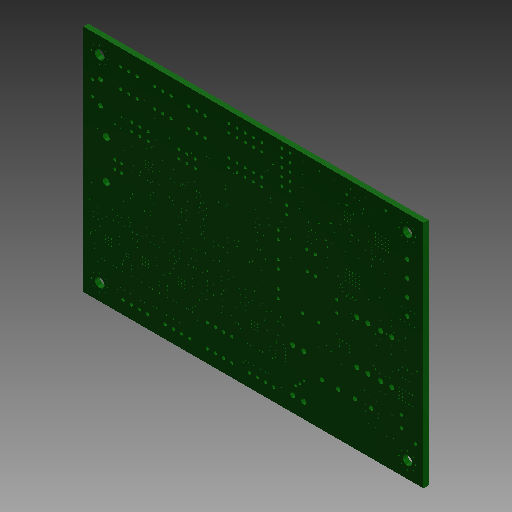
# Autodesk Inventor part: Mini-Rambo_Outline
Saved by Autodesk Inventor 2018.2 (Build 222227000, 227)
## iProperties
Part Number: Mini-Rambo_Outline
Material: Generic
Document SubType Name: Modeling
Designer: autocad
Appearance: Board Outline
Author: autocad
Autodesk Inventor part; units mm, degrees
ref_plane "YZ Plane" through (0, 0, 0) normal (1, 0, 0) x (0, 1, 0)
ref_plane "XZ Plane" through (0, 0, 0) normal (0, 1, 0) x (-1, 0, 0)
ref_plane "XY Plane" through (0, 0, 0) normal (0, 0, 1) x (1, 0, 0)
sketch "Sketch1" plane through (0, 0, 0) normal (0, 0, 1) x (1, 0, 0)
  line L0 (25, 25) -> (25, 96)
  line L1 (25, 96) -> (130, 96)
  line L2 (130, 96) -> (130, 25)
  line L3 (130, 25) -> (25, 25)
  circle A0 centre (93.0018, 43.156) radius 0.8001
  circle A1 centre (89.5982, 43.156) radius 0.8001
  circle A2 centre (89.5982, 29.694) radius 0.8001
  circle A3 centre (93.0018, 29.694) radius 0.8001
  circle A4 centre (109.4232, 60.556) radius 0.8001
  circle A5 centre (112.8268, 60.556) radius 0.8001
  circle A6 centre (112.8268, 47.094) radius 0.8001
  circle A7 centre (109.4232, 47.094) radius 0.8001
  circle A8 centre (116.7982, 47.119) radius 0.8001
  circle A9 centre (120.2018, 47.119) radius 0.8001
  circle A10 centre (120.2018, 60.581) radius 0.8001
  circle A11 centre (116.7982, 60.581) radius 0.8001
  circle A12 centre (69.89, 90.06) radius 0.45
  circle A13 centre (69.89, 92.6) radius 0.45
  circle A14 centre (72.43, 90.06) radius 0.45
  circle A15 centre (72.43, 92.6) radius 0.45
  circle A16 centre (74.97, 90.06) radius 0.45
  circle A17 centre (74.97, 92.6) radius 0.45
  circle A18 centre (77.51, 90.06) radius 0.45
  circle A19 centre (77.51, 92.6) radius 0.45
  circle A20 centre (80.05, 90.06) radius 0.45
  circle A21 centre (80.05, 92.6) radius 0.45
  circle A22 centre (69.84, 80.735) radius 0.45
  circle A23 centre (69.84, 83.275) radius 0.45
  circle A24 centre (72.38, 80.735) radius 0.45
  circle A25 centre (72.38, 83.275) radius 0.45
  circle A26 centre (74.92, 80.735) radius 0.45
  circle A27 centre (74.92, 83.275) radius 0.45
  circle A28 centre (77.46, 80.735) radius 0.45
  circle A29 centre (77.46, 83.275) radius 0.45
  circle A30 centre (80, 80.735) radius 0.45
  circle A31 centre (80, 83.275) radius 0.45
  circle A32 centre (63.19, 29) radius 0.508
  circle A33 centre (65.73, 29) radius 0.508
  circle A34 centre (68.27, 29) radius 0.508
  circle A35 centre (70.81, 29) radius 0.508
  circle A36 centre (63.19, 36) radius 0.508
  circle A37 centre (65.73, 36) radius 0.508
  circle A38 centre (68.27, 36) radius 0.508
  circle A39 centre (70.81, 36) radius 0.508
  circle A40 centre (27.7554, 83.2606) radius 0.508
  circle A41 centre (27.7554, 78.7394) radius 0.508
  circle A42 centre (30.2446, 84.5052) radius 0.7493
  circle A43 centre (30.2446, 77.4948) radius 0.7493
  circle A44 centre (57.46, 91) radius 0.508
  circle A45 centre (60, 91) radius 0.508
  circle A46 centre (62.54, 91) radius 0.508
  circle A47 centre (46.96, 91) radius 0.508
  circle A48 centre (49.5, 91) radius 0.508
  circle A49 centre (52.04, 91) radius 0.508
  circle A50 centre (36.46, 91) radius 0.508
  circle A51 centre (39, 91) radius 0.508
  circle A52 centre (41.54, 91) radius 0.508
  circle A53 centre (52.04, 85) radius 0.508
  circle A54 centre (49.5, 85) radius 0.508
  circle A55 centre (46.96, 85) radius 0.508
  circle A56 centre (62.54, 85) radius 0.508
  circle A57 centre (60, 85) radius 0.508
  circle A58 centre (57.46, 85) radius 0.508
  circle A59 centre (41.54, 85) radius 0.508
  circle A60 centre (39, 85) radius 0.508
  circle A61 centre (36.46, 85) radius 0.508
  circle A62 centre (85.1, 69.13) radius 0.508
  circle A63 centre (85.1, 71.67) radius 0.508
  circle A64 centre (85.1, 61.23) radius 0.508
  circle A65 centre (85.1, 63.77) radius 0.508
  circle A66 centre (87.7, 79.67) radius 0.508
  circle A67 centre (87.7, 77.13) radius 0.508
  circle A68 centre (94.13, 65.1) radius 0.508
  circle A69 centre (96.67, 65.1) radius 0.508
  circle A70 centre (85.1, 53.33) radius 0.508
  circle A71 centre (85.1, 55.87) radius 0.508
  circle A72 centre (88.765, 83.965) radius 0.45
  circle A73 centre (86.225, 83.965) radius 0.45
  circle A74 centre (88.765, 86.505) radius 0.45
  circle A75 centre (86.225, 86.505) radius 0.45
  circle A76 centre (88.765, 89.045) radius 0.45
  circle A77 centre (86.225, 89.045) radius 0.45
  circle A78 centre (88.765, 91.585) radius 0.45
  circle A79 centre (86.225, 91.585) radius 0.45
  circle A80 centre (88.765, 94.125) radius 0.45
  circle A81 centre (86.225, 94.125) radius 0.45
  circle A82 centre (32, 57.9802) radius 1.1049
  circle A83 centre (32, 70) radius 1.1049
  circle A84 centre (34.7178, 62.73) radius 0.4826
  circle A85 centre (34.7178, 65.25) radius 0.4826
  circle A86 centre (36.7244, 65.25) radius 0.4826
  circle A87 centre (36.7244, 62.73) radius 0.4826
  circle A88 centre (97.65, 53.2) radius 0.508
  circle A89 centre (92.65, 53.2) radius 0.508
  circle A90 centre (37.19, 29) radius 0.508
  circle A91 centre (39.73, 29) radius 0.508
  circle A92 centre (42.27, 29) radius 0.508
  circle A93 centre (44.81, 29) radius 0.508
  circle A94 centre (50.19, 29) radius 0.508
  circle A95 centre (52.73, 29) radius 0.508
  circle A96 centre (55.27, 29) radius 0.508
  circle A97 centre (57.81, 29) radius 0.508
  circle A98 centre (76.19, 29) radius 0.508
  circle A99 centre (78.73, 29) radius 0.508
  circle A100 centre (81.27, 29) radius 0.508
  circle A101 centre (83.81, 29) radius 0.508
  circle A102 centre (124.9934, 68.58) radius 0.6985
  circle A103 centre (124.9934, 73.66) radius 0.6985
  circle A104 centre (124.9934, 78.74) radius 0.6985
  circle A105 centre (124.9934, 83.82) radius 0.6985
  circle A106 centre (103.225, 62.103) radius 0.508
  circle A107 centre (103.225, 58.547) radius 0.508
  circle A108 centre (123.15, 37.722) radius 0.508
  circle A109 centre (123.15, 41.278) radius 0.508
  circle A110 centre (54.41, 75.376) radius 0.4826
  circle A111 centre (54.41, 77.916) radius 0.4826
  circle A112 centre (56.95, 75.376) radius 0.4826
  circle A113 centre (56.95, 77.916) radius 0.4826
  circle A114 centre (59.49, 75.376) radius 0.4826
  circle A115 centre (59.49, 77.916) radius 0.4826
  circle A116 centre (39.866, 75.376) radius 0.4826
  circle A117 centre (39.866, 77.916) radius 0.4826
  circle A118 centre (42.406, 75.376) radius 0.4826
  circle A119 centre (42.406, 77.916) radius 0.4826
  circle A120 centre (44.946, 75.376) radius 0.4826
  circle A121 centre (44.946, 77.916) radius 0.4826
  circle A122 centre (94, 70.9) radius 0.508
  circle A123 centre (96.54, 70.9) radius 0.508
  circle A124 centre (127.525, 35.7) radius 0.508
  circle A125 centre (123.222, 28.222) radius 0.1905
  circle A126 centre (126.778, 28.222) radius 0.1905
  circle A127 centre (126.778, 31.778) radius 0.1905
  circle A128 centre (123.222, 31.778) radius 0.1905
  circle A129 centre (122.46, 30) radius 0.1905
  circle A130 centre (127.54, 30) radius 0.1905
  circle A131 centre (125, 32.54) radius 0.1905
  circle A132 centre (125, 27.46) radius 0.1905
  circle A133 centre (28.222, 28.222) radius 0.1905
  circle A134 centre (31.778, 28.222) radius 0.1905
  circle A135 centre (31.778, 31.778) radius 0.1905
  circle A136 centre (28.222, 31.778) radius 0.1905
  circle A137 centre (27.46, 30) radius 0.1905
  circle A138 centre (32.54, 30) radius 0.1905
  circle A139 centre (30, 32.54) radius 0.1905
  circle A140 centre (30, 27.46) radius 0.1905
  circle A141 centre (28.222, 89.222) radius 0.1905
  circle A142 centre (31.778, 89.222) radius 0.1905
  circle A143 centre (31.778, 92.778) radius 0.1905
  circle A144 centre (28.222, 92.778) radius 0.1905
  circle A145 centre (27.46, 91) radius 0.1905
  circle A146 centre (32.54, 91) radius 0.1905
  circle A147 centre (30, 93.54) radius 0.1905
  circle A148 centre (30, 88.46) radius 0.1905
  circle A149 centre (123.222, 89.222) radius 0.1905
  circle A150 centre (126.778, 89.222) radius 0.1905
  circle A151 centre (126.778, 92.778) radius 0.1905
  circle A152 centre (123.222, 92.778) radius 0.1905
  circle A153 centre (122.46, 91) radius 0.1905
  circle A154 centre (127.54, 91) radius 0.1905
  circle A155 centre (125, 93.54) radius 0.1905
  circle A156 centre (125, 88.46) radius 0.1905
  circle A157 centre (98.605, 38.375) radius 0.6985
  circle A158 centre (103.685, 38.375) radius 0.6985
  circle A159 centre (108.765, 38.375) radius 0.6985
  circle A160 centre (113.845, 38.375) radius 0.6985
  circle A161 centre (97.625, 46.375) radius 0.1905
  circle A162 centre (101.45, 47.325) radius 0.1905
  circle A163 centre (99.95, 48.25) radius 0.1905
  circle A164 centre (86.075, 30.1) radius 0.1905
  circle A165 centre (84.375, 39.1) radius 0.1905
  circle A166 centre (84.5, 41.175) radius 0.1905
  circle A167 centre (87.375, 38.5) radius 0.1905
  circle A168 centre (87.375, 41.1437) radius 0.1905
  circle A169 centre (108.025, 59) radius 0.1905
  circle A170 centre (107.9, 60.775) radius 0.1905
  circle A171 centre (93.15, 35.35) radius 0.381
  circle A172 centre (91.775, 33.9) radius 0.381
  circle A173 centre (120.7, 33.775) radius 0.1905
  circle A174 centre (118.525, 33.2) radius 0.1905
  circle A175 centre (87.375, 40.2625) radius 0.1905
  circle A176 centre (87.375, 39.3813) radius 0.1905
  circle A177 centre (87.375, 37.6187) radius 0.1905
  circle A178 centre (125.725, 51.4) radius 0.1905
  circle A179 centre (124.525, 51.4) radius 0.1905
  circle A180 centre (123.5, 51.4) radius 0.1905
  circle A181 centre (95.325, 73.125) radius 0.1905
  circle A182 centre (94.3, 73.125) radius 0.1905
  circle A183 centre (94.45, 75.875) radius 0.1905
  circle A184 centre (96.8, 75.025) radius 0.1905
  circle A185 centre (96.8, 76.8) radius 0.1905
  circle A186 centre (95.425, 76.8) radius 0.1905
  circle A187 centre (94.3, 74.45) radius 0.1905
  circle A188 centre (88.95, 71.2) radius 0.1905
  circle A189 centre (89.05, 66.25) radius 0.1905
  circle A190 centre (99.85, 76.275) radius 0.3175
  circle A191 centre (115.15, 33.825) radius 0.1905
  circle A192 centre (113.075, 33.825) radius 0.1905
  circle A193 centre (112.175, 38.55) radius 0.1905
  circle A194 centre (58.4232, 78.8982) radius 0.1905
  circle A195 centre (71.375, 79.85) radius 0.1905
  circle A196 centre (117.2, 84.851) radius 0.1905
  circle A197 centre (117.2, 85.867) radius 0.1905
  circle A198 centre (117.2, 83.835) radius 0.1905
  circle A199 centre (117.2, 82.819) radius 0.1905
  circle A200 centre (116.184, 82.819) radius 0.1905
  circle A201 centre (115.168, 82.819) radius 0.1905
  circle A202 centre (115.168, 83.835) radius 0.1905
  circle A203 centre (116.184, 83.835) radius 0.1905
  circle A204 centre (116.184, 84.851) radius 0.1905
  circle A205 centre (115.168, 84.851) radius 0.1905
  circle A206 centre (115.168, 85.867) radius 0.1905
  circle A207 centre (116.184, 85.867) radius 0.1905
  circle A208 centre (118.216, 85.867) radius 0.1905
  circle A209 centre (119.232, 85.867) radius 0.1905
  circle A210 centre (119.232, 84.851) radius 0.1905
  circle A211 centre (118.216, 84.851) radius 0.1905
  circle A212 centre (118.216, 83.835) radius 0.1905
  circle A213 centre (119.232, 83.835) radius 0.1905
  circle A214 centre (119.232, 82.819) radius 0.1905
  circle A215 centre (118.216, 82.819) radius 0.1905
  circle A216 centre (109.116, 68.619) radius 0.1905
  circle A217 centre (110.132, 68.619) radius 0.1905
  circle A218 centre (110.132, 69.635) radius 0.1905
  circle A219 centre (109.116, 69.635) radius 0.1905
  circle A220 centre (109.116, 70.651) radius 0.1905
  circle A221 centre (110.132, 70.651) radius 0.1905
  circle A222 centre (110.132, 71.667) radius 0.1905
  circle A223 centre (109.116, 71.667) radius 0.1905
  circle A224 centre (107.084, 71.667) radius 0.1905
  circle A225 centre (106.068, 71.667) radius 0.1905
  circle A226 centre (106.068, 70.651) radius 0.1905
  circle A227 centre (107.084, 70.651) radius 0.1905
  circle A228 centre (107.084, 69.635) radius 0.1905
  circle A229 centre (106.068, 69.635) radius 0.1905
  circle A230 centre (106.068, 68.619) radius 0.1905
  circle A231 centre (107.084, 68.619) radius 0.1905
  circle A232 centre (108.1, 68.619) radius 0.1905
  circle A233 centre (108.1, 69.635) radius 0.1905
  circle A234 centre (108.1, 71.667) radius 0.1905
  circle A235 centre (108.1, 70.651) radius 0.1905
  circle A236 centre (45.212, 68.834) radius 0.1905
  circle A237 centre (45.212, 69.784) radius 0.1905
  circle A238 centre (44.2548, 69.7931) radius 0.1905
  circle A239 centre (44.267, 68.834) radius 0.1905
  circle A240 centre (44.262, 67.859) radius 0.1905
  circle A241 centre (45.212, 67.884) radius 0.1905
  circle A242 centre (46.162, 67.884) radius 0.1905
  circle A243 centre (46.162, 68.834) radius 0.1905
  circle A244 centre (46.162, 69.784) radius 0.1905
  circle A245 centre (32.7, 42.5706) radius 0.1905
  circle A246 centre (31.75, 42.5706) radius 0.1905
  circle A247 centre (31.7409, 41.6134) radius 0.1905
  circle A248 centre (32.7, 41.6256) radius 0.1905
  circle A249 centre (33.675, 41.6206) radius 0.1905
  circle A250 centre (33.65, 42.5706) radius 0.1905
  circle A251 centre (33.65, 43.5206) radius 0.1905
  circle A252 centre (32.7, 43.5206) radius 0.1905
  circle A253 centre (31.75, 43.5206) radius 0.1905
  circle A254 centre (44.153, 42.5706) radius 0.1905
  circle A255 centre (43.203, 42.5706) radius 0.1905
  circle A256 centre (43.1939, 41.6134) radius 0.1905
  circle A257 centre (44.153, 41.6256) radius 0.1905
  circle A258 centre (45.128, 41.6206) radius 0.1905
  circle A259 centre (45.103, 42.5706) radius 0.1905
  circle A260 centre (45.103, 43.5206) radius 0.1905
  circle A261 centre (44.153, 43.5206) radius 0.1905
  circle A262 centre (43.203, 43.5206) radius 0.1905
  circle A263 centre (55.294, 42.5706) radius 0.1905
  circle A264 centre (54.344, 42.5706) radius 0.1905
  circle A265 centre (54.3349, 41.6134) radius 0.1905
  circle A266 centre (55.294, 41.6256) radius 0.1905
  circle A267 centre (56.269, 41.6206) radius 0.1905
  circle A268 centre (56.244, 42.5706) radius 0.1905
  circle A269 centre (56.244, 43.5206) radius 0.1905
  circle A270 centre (55.294, 43.5206) radius 0.1905
  circle A271 centre (54.344, 43.5206) radius 0.1905
  circle A272 centre (77.85, 42.3956) radius 0.1905
  circle A273 centre (76.9, 42.3956) radius 0.1905
  circle A274 centre (76.8909, 41.4384) radius 0.1905
  circle A275 centre (77.85, 41.4506) radius 0.1905
  circle A276 centre (78.825, 41.4456) radius 0.1905
  circle A277 centre (78.8, 42.3956) radius 0.1905
  circle A278 centre (78.8, 43.3456) radius 0.1905
  circle A279 centre (77.85, 43.3456) radius 0.1905
  circle A280 centre (76.9, 43.3456) radius 0.1905
  circle A281 centre (39.1922, 49.6062) radius 0.1905
  circle A282 centre (39.37, 50.927) radius 0.1905
  circle A283 centre (102.5398, 79.7052) radius 0.1905
  circle A284 centre (107.2388, 82.7532) radius 0.1905
  circle A285 centre (109.9566, 81.3816) radius 0.1905
  circle A286 centre (103.6828, 88.011) radius 0.1905
  circle A287 centre (108.3818, 87.5792) radius 0.1905
  circle A288 centre (107.8484, 81.6864) radius 0.3556
  circle A289 centre (111.47, 90.465) radius 0.1905
  circle A290 centre (106.2482, 91.7956) radius 0.381
  circle A291 centre (112.1156, 79.7052) radius 0.1905
  circle A292 centre (107.3277, 79.7052) radius 0.1905
  circle A293 centre (91.694, 80.772) radius 0.1905
  circle A294 centre (97.7519, 79.7052) radius 0.1905
  circle A295 centre (106.239, 88.8896) radius 0.381
  circle A296 centre (82.2198, 31.6992) radius 0.1905
  circle A297 centre (79.7814, 31.6992) radius 0.1905
  circle A298 centre (77.597, 31.6992) radius 0.1905
  circle A299 centre (54.5338, 31.6992) radius 0.1905
  circle A300 centre (35.5092, 30.9372) radius 0.1905
  circle A301 centre (44.3738, 73.0504) radius 0.1905
  circle A302 centre (36.5252, 74.5998) radius 0.1905
  circle A303 centre (51.5112, 79.4512) radius 0.1905
  circle A304 centre (43.942, 85.725) radius 0.1905
  circle A305 centre (62.475, 61.55) radius 0.1905
  circle A306 centre (76.2, 58.675) radius 0.1905
  circle A307 centre (80.425, 49.575) radius 0.1905
  circle A308 centre (60.775, 65.55) radius 0.1905
  circle A309 centre (62.1, 63.075) radius 0.1905
  circle A310 centre (60.45, 64) radius 0.1905
  circle A311 centre (66.5828, 58.325) radius 0.1905
  circle A312 centre (68.7999, 69.7999) radius 0.1905
  circle A313 centre (68.1, 58.6) radius 0.1905
  circle A314 centre (69.3, 57.8) radius 0.1905
  circle A315 centre (69.4999, 60.4999) radius 0.1905
  circle A316 centre (69.5, 61.8) radius 0.1905
  circle A317 centre (69.4981, 70.6784) radius 0.1905
  circle A318 centre (27.2, 41.9) radius 0.1905
  circle A319 centre (90.5, 32.7) radius 0.381
  circle A320 centre (84.375, 38.1875) radius 0.1905
  circle A321 centre (84.375, 37.275) radius 0.1905
  circle A322 centre (107.225, 50.075) radius 0.1905
  circle A323 centre (107.225, 50.975) radius 0.1905
  circle A324 centre (107.225, 51.875) radius 0.1905
  circle A325 centre (106.1583, 51.875) radius 0.1905
  circle A326 centre (105.0917, 51.875) radius 0.1905
  circle A327 centre (104.025, 51.875) radius 0.1905
  circle A328 centre (104.025, 50.975) radius 0.1905
  circle A329 centre (104.025, 50.075) radius 0.1905
  circle A330 centre (124.525, 45.2) radius 0.1905
  circle A331 centre (123.5, 45.2) radius 0.1905
  circle A332 centre (122.475, 45.2) radius 0.1905
  circle A333 centre (126.575, 45.2) radius 0.1905
  circle A334 centre (124.525, 48.3) radius 0.1905
  circle A335 centre (80, 58.2) radius 0.1905
  circle A336 centre (77.2, 59.425) radius 0.1905
  circle A337 centre (122.475, 47.2) radius 0.1905
  circle A338 centre (122.475, 48.2) radius 0.1905
  circle A339 centre (123.5, 48.25) radius 0.1905
  circle A340 centre (125.55, 48.25) radius 0.1905
  circle A341 centre (126.575, 48.25) radius 0.1905
  circle A342 centre (125.55, 45.2) radius 0.1905
  circle A343 centre (122.475, 46.2) radius 0.1905
  circle A344 centre (103.075, 52.925) radius 0.1905
  circle A345 centre (101.3218, 81.5936) radius 0.381
  circle A346 centre (111.125, 89.154) radius 0.1905
  circle A347 centre (118.3, 93.5) radius 0.3556
  circle A348 centre (106.8, 65.2) radius 0.1905
  circle A349 centre (104.2, 65.7) radius 0.1905
  circle A350 centre (104.2, 66.7) radius 0.1905
  circle A351 centre (105.1, 65.2) radius 0.1905
  circle A352 centre (105.1, 67.2) radius 0.1905
  circle A353 centre (105.1, 66.2) radius 0.1905
  circle A354 centre (106.2, 64.6) radius 0.1905
  circle A355 centre (107.5, 64.6) radius 0.1905
  circle A356 centre (109.3, 65.2) radius 0.1905
  circle A357 centre (108.7, 64.6) radius 0.1905
  circle A358 centre (108.1, 65.2) radius 0.1905
  circle A359 centre (117.8, 79.6) radius 0.1905
  circle A360 centre (116.6, 79.6) radius 0.1905
  circle A361 centre (115.3, 79.6) radius 0.1905
  circle A362 centre (114.1, 79.8) radius 0.1905
  circle A363 centre (114.1, 80.6) radius 0.1905
  circle A364 centre (114.1, 81.4) radius 0.1905
  circle A365 centre (112.9, 67) radius 0.1905
  circle A366 centre (113.4618, 41.148) radius 0.1905
  circle A367 centre (115.6, 41) radius 0.1905
  circle A368 centre (116.2, 38.1) radius 0.1905
  circle A369 centre (115.975, 36.8) radius 0.1905
  circle A370 centre (112.175, 36.75) radius 0.1905
  circle A371 centre (111.9, 42.2) radius 0.1905
  circle A372 centre (120.3, 39.8) radius 0.1905
  circle A373 centre (118.1608, 44.1198) radius 0.1905
  circle A374 centre (116.5606, 44.1198) radius 0.1905
  circle A375 centre (119.4562, 49.3776) radius 0.1905
  circle A376 centre (118.3894, 49.022) radius 0.1905
  circle A377 centre (116.3574, 49.022) radius 0.1905
  circle A378 centre (115.2144, 49.53) radius 0.1905
  circle A379 centre (120.523, 51.4096) radius 0.1905
  circle A380 centre (114.5032, 50.1904) radius 0.1905
  circle A381 centre (128.025, 55.25) radius 0.1905
  circle A382 centre (123.6, 54.2) radius 0.1905
  circle A383 centre (125, 54.2) radius 0.1905
  circle A384 centre (122.3, 52.8) radius 0.1905
  circle A385 centre (120.65, 61.976) radius 0.1905
  circle A386 centre (116.84, 63.2714) radius 0.1905
  circle A387 centre (120.2, 58.175) radius 0.1905
  circle A388 centre (116.75, 58.1) radius 0.1905
  circle A389 centre (115.2, 58.85) radius 0.1905
  circle A390 centre (97.8535, 93.8022) radius 0.1905
  circle A391 centre (104.4702, 82.804) radius 0.254
  circle A392 centre (93.0656, 93.8022) radius 0.1905
  circle A393 centre (102.6414, 93.8022) radius 0.1905
  circle A394 centre (107.4293, 93.8022) radius 0.1905
  circle A395 centre (112.2172, 93.8022) radius 0.1905
  circle A396 centre (114.3, 78.5) radius 0.1905
  circle A397 centre (113.157, 82.6008) radius 0.1905
  circle A398 centre (92.5322, 86.6648) radius 0.1905
  circle A399 centre (92.5322, 82.9564) radius 0.1905
  circle A400 centre (113.157, 86.6521) radius 0.1905
  circle A401 centre (94.5, 78.5) radius 0.1905
  circle A402 centre (92.5322, 90.3732) radius 0.1905
  circle A403 centre (110.1852, 92.1512) radius 0.1905
  circle A404 centre (108.7008, 92.1824) radius 0.1905
  circle A405 centre (113.157, 90.7034) radius 0.1905
  circle A406 centre (39.75, 38.5) radius 0.1905
  circle A407 centre (28.4734, 38.3032) radius 0.1905
  circle A408 centre (37, 38.5) radius 0.1905
  circle A409 centre (51, 38.5) radius 0.1905
  circle A410 centre (48.5, 38.5) radius 0.1905
  circle A411 centre (73.5, 39.5) radius 0.1905
  circle A412 centre (83.439, 36.576) radius 0.1905
  circle A413 centre (81, 45.5) radius 0.1905
  circle A414 centre (75.184, 45.085) radius 0.1905
  circle A415 centre (58.5, 45.5) radius 0.1905
  circle A416 centre (52.705, 45.212) radius 0.1905
  circle A417 centre (47.5, 45.5) radius 0.1905
  circle A418 centre (41.529, 45.212) radius 0.1905
  circle A419 centre (36, 45.5) radius 0.1905
  circle A420 centre (30.099, 45.212) radius 0.1905
  circle A421 centre (83.225, 48.875) radius 0.1905
  circle A422 centre (72.9, 62.575) radius 0.1905
  circle A423 centre (81.675, 43.15) radius 0.1905
  circle A424 centre (82.8, 39.4) radius 0.1905
  circle A425 centre (37.175, 39.625) radius 0.1905
  circle A426 centre (39.7, 39.6) radius 0.1905
  circle A427 centre (50.9, 39.6) radius 0.1905
  circle A428 centre (48.5, 39.6) radius 0.1905
  circle A429 centre (35.9, 49) radius 0.1905
  circle A430 centre (28.425, 39.6) radius 0.1905
  circle A431 centre (72.8, 40.4) radius 0.1905
  circle A432 centre (84.5, 41.8) radius 0.1905
  circle A433 centre (38.9, 41.975) radius 0.1905
  circle A434 centre (50.1, 41.9) radius 0.1905
  circle A435 centre (79.7, 48.8) radius 0.1905
  circle A436 centre (81.5, 48) radius 0.1905
  circle A437 centre (79.3, 36.6) radius 0.1905
  circle A438 centre (76.5, 36.6) radius 0.1905
  circle A439 centre (80.2, 36.6) radius 0.1905
  circle A440 centre (75.6, 36.6) radius 0.1905
  circle A441 centre (47.575, 43.325) radius 0.1905
  circle A442 centre (46, 74.1) radius 0.1905
  circle A443 centre (52.725, 71.725) radius 0.1905
  circle A444 centre (51.95, 68.775) radius 0.1905
  circle A445 centre (39.925, 64.3) radius 0.1905
  circle A446 centre (40.525, 66.575) radius 0.1905
  circle A447 centre (43.825, 56.075) radius 0.1905
  circle A448 centre (42.175, 64.85) radius 0.1905
  circle A449 centre (39.5, 57.35) radius 0.1905
  circle A450 centre (63.9781, 80.2539) radius 0.1905
  circle A451 centre (62.2, 67.6) radius 0.1905
  circle A452 centre (61.253, 68.5783) radius 0.1905
  circle A453 centre (72.425, 60.85) radius 0.1905
  circle A454 centre (81.9, 73.15) radius 0.1905
  circle A455 centre (59.35, 71.725) radius 0.1905
  circle A456 centre (62.75, 54.325) radius 0.1905
  circle A457 centre (59.9029, 53.5276) radius 0.1905
  circle A458 centre (69.7, 53.25) radius 0.1905
  circle A459 centre (71.3038, 52.275) radius 0.1905
  circle A460 centre (71.75, 62.25) radius 0.1905
  circle A461 centre (59.6, 50.7331) radius 0.1905
  circle A462 centre (79.35, 70.325) radius 0.1905
  circle A463 centre (56.55, 69.275) radius 0.1905
  circle A464 centre (47, 82.4) radius 0.1905
  circle A465 centre (69.025, 47.625) radius 0.1905
  circle A466 centre (46.675, 74.8) radius 0.1905
  circle A467 centre (67.6, 40.9) radius 0.1905
  circle A468 centre (63.2, 45.8) radius 0.1905
  circle A469 centre (63.25, 47.125) radius 0.1905
  circle A470 centre (67.8, 42.6) radius 0.1905
  circle A471 centre (71.825, 44.275) radius 0.1905
  circle A472 centre (67.6, 45.8) radius 0.1905
  circle A473 centre (45.7772, 48.7274) radius 0.1905
  circle A474 centre (29.21, 50.165) radius 0.1905
  circle A475 centre (48.5, 48.7) radius 0.1905
  circle A476 centre (47.1, 48.7) radius 0.1905
  circle A477 centre (34.25, 36.725) radius 0.1905
  circle A478 centre (31.325, 36.7) radius 0.1905
  circle A479 centre (37.719, 48.8442) radius 0.1905
  circle A480 centre (30.5, 36.7) radius 0.1905
  circle A481 centre (52.9, 36.6) radius 0.1905
  circle A482 centre (36.2544, 43.3206) radius 0.1905
  circle A483 centre (60.9, 40.8) radius 0.1905
  circle A484 centre (27.5, 42.5) radius 0.1905
  circle A485 centre (49.4, 41.9) radius 0.1905
  circle A486 centre (55.2527, 61.503) radius 0.1905
  circle A487 centre (54.9, 68.4) radius 0.1905
  circle A488 centre (79.6, 63.6) radius 0.1905
  circle A489 centre (48.5774, 65.4282) radius 0.1905
  circle A490 centre (49.4716, 72.3179) radius 0.1905
  circle A491 centre (63.225, 44.5) radius 0.1905
  circle A492 centre (45.825, 56.925) radius 0.1905
  circle A493 centre (45.825, 55.95) radius 0.1905
  circle A494 centre (37.8, 77.7) radius 0.1905
  circle A495 centre (40.15, 71.5) radius 0.1905
  circle A496 centre (48.575, 69.1) radius 0.1905
  circle A497 centre (82.3, 71.6) radius 0.1905
  circle A498 centre (78.8, 71.5) radius 0.1905
  circle A499 centre (78.5998, 65.4999) radius 0.1905
  circle A500 centre (78.2, 70.1) radius 0.1905
  circle A501 centre (65.125, 44.325) radius 0.1905
  circle A502 centre (68.1, 44.5) radius 0.1905
  circle A503 centre (65.125, 47.1) radius 0.1905
  circle A504 centre (58.8, 43.325) radius 0.1905
  circle A505 centre (38.125, 41.95) radius 0.1905
  circle A506 centre (51.725, 43.325) radius 0.1905
  circle A507 centre (40.125, 58.775) radius 0.1905
  circle A508 centre (32.258, 48.768) radius 0.1905
  circle A509 centre (34.3, 48.875) radius 0.1905
  circle A510 centre (78.5998, 63.2999) radius 0.1905
  circle A511 centre (57, 70.3) radius 0.1905
  circle A512 centre (58.925, 48.725) radius 0.1905
  circle A513 centre (55.4, 57.1) radius 0.1905
  circle A514 centre (52.4, 63.275) radius 0.1905
  circle A515 centre (55.6, 69.2) radius 0.1905
  circle A516 centre (52.9124, 62.3876) radius 0.1905
  circle A517 centre (51.6, 63.7) radius 0.1905
  circle A518 centre (51.4376, 66.645) radius 0.1905
  circle A519 centre (53.1926, 68.4) radius 0.1905
  circle A520 centre (54.61, 57.9374) radius 0.1905
  circle A521 centre (55.3574, 56.1426) radius 0.1905
  circle A522 centre (35.4182, 50.8) radius 0.1905
  circle A523 centre (65.225, 53.525) radius 0.1905
  circle A524 centre (66.975, 54.325) radius 0.1905
  circle A525 centre (67.7, 50.5) radius 0.1905
  circle A526 centre (44.5008, 51.9176) radius 0.1905
  circle A527 centre (44.5262, 49.8856) radius 0.1905
  circle A528 centre (36.8, 50.8) radius 0.1905
  circle A529 centre (58.85, 53.575) radius 0.1905
  circle A530 centre (68.0783, 47.0273) radius 0.1905
  circle A531 centre (67.7, 49.5) radius 0.1905
  circle A532 centre (59.9, 48.7) radius 0.1905
  circle A533 centre (63.2531, 49.7524) radius 0.1905
  circle A534 centre (55.9027, 54.0276) radius 0.1905
  circle A535 centre (57.3532, 48.6918) radius 0.1905
  circle A536 centre (58.2168, 50.5968) radius 0.1905
  circle A537 centre (78.2038, 73.6962) radius 0.1905
  circle A538 centre (70.8, 41.6) radius 0.1905
  circle A539 centre (72.1, 40.4) radius 0.1905
  circle A540 centre (28.775, 43.3206) radius 0.1905
  circle A541 centre (54.483, 48.768) radius 0.1905
  circle A542 centre (78.6, 67.8) radius 0.1905
  circle A543 centre (78.2, 68.85) radius 0.1905
  circle A544 centre (68.8784, 75.4787) radius 0.1905
  circle A545 centre (55.1474, 60.4774) radius 0.1905
  circle A546 centre (61.075, 60.525) radius 0.1905
  circle A547 centre (55.3, 62.5) radius 0.1905
  circle A548 centre (62.875, 64.35) radius 0.1905
  circle A549 centre (57.0142, 65.3) radius 0.1905
  circle A550 centre (56.6778, 60.1029) radius 0.1905
  circle A551 centre (57.404, 55.5752) radius 0.1905
  circle A552 centre (61.375, 58.725) radius 0.1905
  circle A553 centre (56.6778, 62.703) radius 0.1905
  circle A554 centre (62.2, 59.775) radius 0.1905
  circle A555 centre (59.8999, 69.4999) radius 0.1905
  circle A556 centre (59.7999, 67.6999) radius 0.1905
  circle A557 centre (61.1, 66.9) radius 0.1905
  circle A558 centre (62.475, 58.05) radius 0.1905
  circle A559 centre (65.3032, 57.3278) radius 0.1905
  circle A560 centre (62.85, 66.35) radius 0.1905
  circle A561 centre (66.6783, 69.9034) radius 0.1905
  circle A562 centre (60.8397, 69.4941) radius 0.1905
  circle A563 centre (65.25, 58.6) radius 0.1905
  circle A564 centre (62.025, 65.3) radius 0.1905
  circle A565 centre (86.2, 74.5) radius 0.1905
  circle A566 centre (122.775, 66.675) radius 0.1905
  circle A567 centre (124.2333, 66.675) radius 0.1905
  circle A568 centre (127.2, 70.3) radius 0.1905
  circle A569 centre (127.15, 66.675) radius 0.1905
  circle A570 centre (124.6, 70.3) radius 0.1905
  circle A571 centre (123.3, 70.3) radius 0.1905
  circle A572 centre (125.9, 70.3) radius 0.1905
  circle A573 centre (125.6917, 66.675) radius 0.1905
  circle A574 centre (34.65, 74.75) radius 0.3556
  circle A575 centre (30.988, 47.625) radius 0.1905
  circle A576 centre (29.464, 46.736) radius 0.1905
  circle A577 centre (29.464, 48.133) radius 0.1905
  circle A578 centre (28.194, 48.133) radius 0.1905
  circle A579 centre (28.194, 46.736) radius 0.1905
  circle A580 centre (43.307, 48.895) radius 0.1905
  circle A581 centre (42.418, 47.625) radius 0.1905
  circle A582 centre (53.594, 47.625) radius 0.1905
  circle A583 centre (40.132, 46.863) radius 0.1905
  circle A584 centre (41.529, 46.863) radius 0.1905
  circle A585 centre (41.529, 48.641) radius 0.1905
  circle A586 centre (40.132, 48.641) radius 0.1905
  circle A587 centre (51.562, 46.736) radius 0.1905
  circle A588 centre (52.959, 46.736) radius 0.1905
  circle A589 centre (51.562, 48.641) radius 0.1905
  circle A590 centre (52.959, 48.641) radius 0.1905
  circle A591 centre (77.216, 48.895) radius 0.1905
  circle A592 centre (75.946, 47.752) radius 0.1905
  circle A593 centre (73.533, 48.641) radius 0.1905
  circle A594 centre (75.184, 48.641) radius 0.1905
  circle A595 centre (75.184, 46.482) radius 0.1905
  circle A596 centre (73.533, 46.482) radius 0.1905
  circle A597 centre (85.09, 47.117) radius 0.1905
  circle A598 centre (85.852, 48.768) radius 0.1905
  circle A599 centre (85.09, 43.561) radius 0.1905
  circle A600 centre (86.614, 41.91) radius 0.1905
  circle A601 centre (86.614, 46.99) radius 0.1905
  circle A602 centre (80.391, 55.372) radius 0.1905
  circle A603 centre (81.28, 61.976) radius 0.1905
  circle A604 centre (80.518, 67.945) radius 0.1905
  circle A605 centre (77.8002, 51.7398) radius 0.1905
  circle A606 centre (74.93, 50.8) radius 0.1905
  circle A607 centre (73.1082, 49.9942) radius 0.1905
  circle A608 centre (69.85, 50.8) radius 0.1905
  circle A609 centre (61.849, 48.641) radius 0.1905
  circle A610 centre (54.737, 50.8) radius 0.1905
  circle A611 centre (52.705, 50.165) radius 0.1905
  circle A612 centre (49.276, 51.435) radius 0.1905
  circle A613 centre (46.736, 50.8) radius 0.1905
  circle A614 centre (33.782, 51.562) radius 0.1905
  circle A615 centre (26.924, 50.8) radius 0.1905
  circle A616 centre (44.65, 64.675) radius 0.1905
  circle A617 centre (45.8, 60.3) radius 0.1905
  circle A618 centre (45.775, 61.3) radius 0.1905
  circle A619 centre (46.736, 59.182) radius 0.1905
  circle A620 centre (54.356, 59.6138) radius 0.1905
  circle A621 centre (46.5074, 62.4586) radius 0.1905
  circle A622 centre (45.6438, 64.6938) radius 0.1905
  circle A623 centre (46.4566, 65.3034) radius 0.1905
  circle A624 centre (38.1, 67.1322) radius 0.1905
  circle A625 centre (37.3888, 68.961) radius 0.1905
  circle A626 centre (38.8874, 51.816) radius 0.1905
  circle A627 centre (49.784, 50.546) radius 0.1905
  circle A628 centre (82.5, 38) radius 0.1905
  circle A629 centre (36.4998, 31.9532) radius 0.1905
  circle A630 centre (75.1078, 31.6992) radius 0.1905
  circle A631 centre (35.1, 36.7) radius 0.1905
  circle A632 centre (37, 36.5) radius 0.1905
  circle A633 centre (29.3624, 35.3822) radius 0.1905
  circle A634 centre (53.7, 36.6) radius 0.1905
  circle A635 centre (52.8574, 31.6992) radius 0.1905
  circle A636 centre (74.2442, 30.8864) radius 0.1905
  circle A637 centre (60.2996, 35.1028) radius 0.1905
  circle A638 centre (56.7, 36.5) radius 0.1905
  circle A639 centre (57.5, 36.5) radius 0.1905
  circle A640 centre (61.5442, 42.7482) radius 0.1905
  circle A641 centre (58.801, 37.719) radius 0.1905
  circle A642 centre (58.6232, 36.4998) radius 0.1905
  circle A643 centre (42.545, 31.623) radius 0.1905
  circle A644 centre (50.5714, 31.6738) radius 0.1905
  circle A645 centre (42.8, 36.6) radius 0.1905
  circle A646 centre (46.3, 36.5) radius 0.1905
  circle A647 centre (51, 36.5) radius 0.1905
  circle A648 centre (43.815, 31.6992) radius 0.1905
  circle A649 centre (46.6852, 32.004) radius 0.1905
  circle A650 centre (45.5, 36.5) radius 0.1905
  circle A651 centre (39.75, 36.5) radius 0.1905
  circle A652 centre (41.8, 36.6) radius 0.1905
  circle A653 centre (37.7698, 31.877) radius 0.1905
  circle A654 centre (62.865, 42.0624) radius 0.1905
  circle A655 centre (59.69, 38.5572) radius 0.1905
  circle A656 centre (47.5742, 31.9786) radius 0.1905
  circle A657 centre (48.5, 36.5) radius 0.1905
  circle A658 centre (39.3954, 31.9278) radius 0.1905
  circle A659 centre (76.073, 31.6738) radius 0.1905
  circle A660 centre (81.2546, 31.6992) radius 0.1905
  circle A661 centre (38.125, 41.2) radius 0.1905
  circle A662 centre (38.9, 41.2) radius 0.1905
  circle A663 centre (105.545, 84.765) radius 0.1905
  circle A664 centre (106.545, 84.765) radius 0.1905
  circle A665 centre (107.545, 84.765) radius 0.1905
  circle A666 centre (107.545, 85.765) radius 0.1905
  circle A667 centre (107.545, 86.765) radius 0.1905
  circle A668 centre (106.545, 86.765) radius 0.1905
  circle A669 centre (105.545, 86.765) radius 0.1905
  circle A670 centre (105.545, 85.765) radius 0.1905
  circle A671 centre (106.545, 85.765) radius 0.1905
  circle A672 centre (87.5, 73.5) radius 0.1905
  circle A673 centre (82.825, 79.05) radius 0.1905
  circle A674 centre (82.825, 77.875) radius 0.1905
  circle A675 centre (68.9, 74.5) radius 0.1905
  circle A676 centre (83.525, 88.4) radius 0.1905
  circle A677 centre (62.95, 80.325) radius 0.1905
  circle A678 centre (81, 85.1044) radius 0.1905
  circle A679 centre (81.75, 85.85) radius 0.1905
  circle A680 centre (104.675, 45.45) radius 0.1905
  circle A681 centre (123.5, 46.2) radius 0.1905
  circle A682 centre (123.5, 47.2) radius 0.1905
  circle A683 centre (126.425, 53.875) radius 0.1905
  circle A684 centre (118.525, 60.6) radius 0.1905
  circle A685 centre (120.2, 63.3) radius 0.1905
  circle A686 centre (122.175, 60.6) radius 0.1905
  circle A687 centre (115.375, 56.025) radius 0.1905
  circle A688 centre (119.975, 55.9) radius 0.1905
  circle A689 centre (124.375, 59) radius 0.1905
  circle A690 centre (124.525, 62.475) radius 0.1905
  circle A691 centre (120.25, 64.975) radius 0.1905
  circle A692 centre (102, 76.4) radius 0.1905
  circle A693 centre (100.325, 74.7) radius 0.1905
  circle A694 centre (100.4, 69.3) radius 0.1905
  circle A695 centre (103.6, 68.575) radius 0.1905
  circle A696 centre (116.375, 69.325) radius 0.1905
  circle A697 centre (117.9, 72.45) radius 0.1905
  circle A698 centre (117.9, 76.4) radius 0.1905
  circle A699 centre (105.975, 76.4) radius 0.1905
  circle A700 centre (109.95, 76.4) radius 0.1905
  circle A701 centre (113.925, 76.4) radius 0.1905
  circle A702 centre (100.325, 71.85) radius 0.1905
  circle A703 centre (42.55, 65.925) radius 0.1905
  circle A704 centre (47.7, 77.125) radius 0.1905
  circle A705 centre (36.75, 77.725) radius 0.1905
  circle A706 centre (37.275, 55.5) radius 0.1905
  circle A707 centre (27.375, 55.55) radius 0.1905
  circle A708 centre (29.275, 70.975) radius 0.1905
  circle A709 centre (125, 30) radius 1.5
  circle A710 centre (30, 30) radius 1.5
  circle A711 centre (30, 91) radius 1.5
  circle A712 centre (125, 91) radius 1.5
  constraints: 713 centre point, 8 end point
extrude "Mini-Rambo_Outline" add sketch "Sketch1" along normal blind 1.57
body "Solid1"
